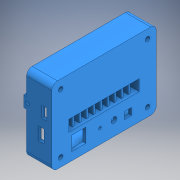
# Autodesk Inventor part: case_front
Saved by Autodesk Inventor 2016 (Build 200138000, 138)
## iProperties
Created: 2018-08-02
Part Number: case_front
Material: Generic
Document SubType Name: Modeling
Designer: Luke
Density: 1 g/cm^3
Appearance: Cyan
Author: Luke
Autodesk Inventor part; units mm, degrees
ref_plane "YZ Plane" through (0, 0, 0) normal (1, 0, 0) x (0, 1, 0)
ref_plane "XZ Plane" through (0, 0, 0) normal (0, 1, 0) x (-1, 0, 0)
ref_plane "XY Plane" through (0, 0, 0) normal (0, 0, 1) x (1, 0, 0)
sketch "Sketch1" plane through (0, 0, 0) normal (0, 1, 0) x (-1, 0, 0)
  line L0 (0, 0) -> (-74.5, 0)
  line L1 (-74.5, 0) -> (-74.5, 54.5)
  line L2 (-74.5, 54.5) -> (0, 54.5)
  line L3 (0, 54.5) -> (0, 0)
  dimension "d0" = 74.5
  dimension "d1" = 54.5
  constraints: 8 end point, 2 parallel, 1 horizontal, 1 perpendicular
  measures "d0" distance of L0.start L0.end
  measures "d1" distance of L0.end L1.end
extrude "Extrusion1" add sketch "Sketch1" along normal blind 2
ref_plane "Work Plane1" through (74.5, 0, 27.25) normal (0, 0, -1) x (-1, 0, 0)
ref_plane "Work Plane2" through (37.25, 0, 54.5) normal (1, 0, 0) x (0, 0, -1)
sketch "Sketch3" plane through (0, 2, 0) normal (0, 1, 0) x (1, 0, 0)
  line L0 (37.25, 10.9) -> (37.25, -65.4) construction
  line L1 (-14.9, -27.25) -> (89.4, -27.25) construction
  circle A0 centre (6.25, -6.25) radius 1.6
  circle A1 centre (68.25, -6.25) radius 1.6
  circle A2 centre (68.25, -48.25) radius 1.6
  circle A3 centre (6.25, -48.25) radius 1.6
  line L2 (6.25, -6.25) -> (68.25, -6.25) construction
  line L3 (68.25, -6.25) -> (68.25, -48.25) construction
  line L4 (68.25, -48.25) -> (6.25, -48.25) construction
  line L5 (6.25, -48.25) -> (6.25, -6.25) construction
  point P0 (0, 0)
  dimension "d4" = 3.2
  dimension "d5" = 3.2
  dimension "d6" = 3.2
  dimension "d7" = 3.2
  dimension "d8" = 62
  dimension "d9" = 42
  constraints: 8 end point, 4 centre point, 4 coincident, 2 parallel, 1 horizontal, 1 perpendicular, 2 other
  measures "d4" diameter of A0
  measures "d5" diameter of A1
  measures "d6" diameter of A2
  measures "d7" diameter of A3
  measures "d8" distance of L2.start L2.end
  measures "d9" distance of L2.end L3.end
extrude "Extrusion2" cut sketch "Sketch3" against normal up to surface (2 mm away)
sketch "Sketch4" plane through (0, 0, 0) normal (0, -1, 0) x (1, 0, 0)
  line L0 (0, 0) -> (74.5, 0) projected
  line L1 (74.5, 0) -> (74.5, 54.5) projected
  line L2 (74.5, 54.5) -> (0, 54.5) projected
  line L3 (0, 54.5) -> (0, 0) projected
  line L4 (72.5, 2) -> (2, 2)
  line L5 (2, 2) -> (2, 52.5)
  line L6 (2, 52.5) -> (72.5, 52.5)
  line L7 (72.5, 52.5) -> (72.5, 2)
  dimension "d12" = 2
  constraints: 8 end point, 3 other
  measures "d12" distance between parallel lines of L4 L0
extrude "Extrusion3" add sketch "Sketch4" along normal blind 16
sketch "Sketch5" plane through (0, 2, 0) normal (0, 1, 0) x (1, 0, 0)
  circle A0 centre (6.25, -48.25) radius 1.6 construction
  line L0 (14.175, -38.675) -> (24.175, -38.675)
  line L1 (24.175, -38.675) -> (24.175, -48.675)
  line L2 (24.175, -48.675) -> (14.175, -48.675)
  line L3 (14.175, -48.675) -> (14.175, -38.675)
  point P0 (0, 0)
  dimension "d15" = 7.925
  dimension "d16" = 10
  dimension "d17" = 10
  dimension "d18" = 9.575
  constraints: 8 end point, 2 parallel, 1 horizontal, 1 perpendicular
  measures "d15" distance from line of A0.centre L3
  measures "d16" distance of L1.end L2.end
  measures "d17" distance of L0.end L1.end
  measures "d18" distance from line of A0.centre L0
extrude "Extrusion4" cut sketch "Sketch5" against normal up to surface (2 mm away)
sketch "Sketch6" plane through (0, 2, 0) normal (-1, 0, 0) x (0, 0, 1)
  line L0 (16.5, -3.5) -> (24.5, -3.5)
  line L1 (24.5, -3.5) -> (24.5, -7)
  line L2 (24.5, -7) -> (16.5, -7)
  line L3 (16.5, -7) -> (16.5, -3.5)
  line L4 (0, 0) -> (54.5, 0) construction
  line L5 (54.5, 0) -> (54.5, -18) construction
  point P0 (0, -2)
  dimension "d21" = 30
  dimension "d22" = 3.5
  dimension "d23" = 8
  dimension "d24" = 3.5
  constraints: 8 end point, 2 parallel, 1 horizontal, 1 perpendicular
  measures "d21" distance between parallel lines of L5 L1
  measures "d22" distance of L0.end L1.end
  measures "d23" distance of L0.start L0.end
  measures "d24" distance between parallel lines of L0 L4
extrude "Extrusion5" cut sketch "Sketch6" against normal up to surface (2 mm away)
sketch "Sketch7" plane through (0, 2, 0) normal (-1, 0, 0) x (0, 0, 1)
  line L0 (0, 0) -> (54.5, 0) construction
  line L1 (54.5, 0) -> (54.5, -18) construction
  line L2 (30.5, -5.5) -> (39.5, -5.5)
  line L3 (39.5, -5.5) -> (39.5, -9.5)
  line L4 (39.5, -9.5) -> (30.5, -9.5)
  line L5 (30.5, -9.5) -> (30.5, -5.5)
  point P0 (0, -2)
  dimension "d27" = 15
  dimension "d28" = 9
  dimension "d29" = 4
  dimension "d30" = 5.5
  constraints: 8 end point, 2 parallel, 1 horizontal, 1 perpendicular
  measures "d27" distance between parallel lines of L1 L3
  measures "d28" distance of L2.start L2.end
  measures "d29" distance of L4.end L2.start
  measures "d30" distance between parallel lines of L2 L0
extrude "Extrusion6" cut sketch "Sketch7" against normal up to surface (2 mm away)
fillet "Fillet1" radius 4 8 edges at (72.5, -8, 52.5) (74.5, -7, 54.5) (72.5, -8, 2) (74.5, -7, 0) (2, -8, 2) (0, -7, 0) (0, -7, 54.5) (2, -8, 52.5)
sketch "Sketch8" plane through (0, -16, 50.5) normal (-1, 0, 0) x (0, 0, 1)
  line L0 (-50.5, 18) -> (-50.5, 0) construction
  line L1 (0, 0) -> (-46.5, 0) construction
  line L2 (-2, 0) -> (-44.5, 0) projected
  line L3 (-26, 0) -> (-34, 0)
  line L4 (-34, 0) -> (-34, -2)
  line L5 (-34, -2) -> (-26, -2)
  line L6 (-26, -2) -> (-26, 0)
  line L7 (-30, -2) -> (-30, 0) construction
  point P0 (-50.5, 16)
  dimension "d34" = 20.5
  dimension "d35" = 8
  dimension "d36" = 2
  constraints: 10 end point, 2 midpoint, 2 parallel, 1 horizontal, 1 perpendicular, 1 point on line
  measures "d34" distance between parallel lines of L0 L7
  measures "d35" distance of L4.end L5.end
  measures "d36" distance of L3.end L4.end
extrude "Extrusion7" add sketch "Sketch8" against normal up to surface (2 mm away)
sketch "Sketch9" plane through (0, -16, 50.5) normal (-1, 0, 0) x (0, 0, 1)
  line L0 (0, 0) -> (-26, 0) construction
  line L1 (-50.5, 18) -> (-50.5, 0) construction
  circle A0 centre (-30, 0.75) radius 1.25
  point P0 (-50.5, 16)
  dimension "d39" = 2.5
  dimension "d43" = 0.75
  dimension "d44" = 20.5
  constraints: 1 centre point
  measures "d39" diameter of A0
  measures "d43" distance from line of A0.centre L0
  measures "d44" distance from line of L1 A0.centre
extrude "Extrusion8" cut sketch "Sketch9" against normal up to surface (2 mm away)
sketch "Sketch10" plane through (0, 2, 0) normal (0, 1, 0) x (1, 0, 0)
  circle A0 centre (6.25, -48.25) radius 1.6 projected
  circle A1 centre (68.25, -48.25) radius 1.6 projected
  line L0 (12.25, -27.75) -> (62.25, -27.75)
  line L1 (62.25, -27.75) -> (62.25, -35.75)
  line L2 (62.25, -35.75) -> (12.25, -35.75)
  line L3 (12.25, -35.75) -> (12.25, -27.75)
  line L4 (6.25, -48.25) -> (68.25, -48.25) construction
  line L5 (37.25, -48.25) -> (37.25, -35.75) construction
  point P0 (0, 0)
  dimension "d45" = 12.5
  dimension "d46" = 8
  dimension "d47" = 50
  constraints: 12 end point, 2 horizontal, 2 midpoint, 2 parallel, 2 perpendicular
  measures "d45" distance from line of L4.start L2
  measures "d46" distance of L2.end L0.start
  measures "d47" distance of L0.start L0.end
extrude "Extrusion9" cut sketch "Sketch10" against normal up to surface (2 mm away) contours L0 L1 L2 L3
sketch "Sketch11" plane through (0, 0, 0) normal (0, -1, 0) x (1, 0, 0)
  line L0 (62.25, 27.75) -> (12.25, 27.75) projected
  line L1 (12.25, 27.75) -> (12.25, 35.75) projected
  line L2 (12.25, 35.75) -> (62.25, 35.75) projected
  line L3 (62.25, 35.75) -> (62.25, 27.75) projected
  line L4 (63.75, 37.25) -> (10.75, 37.25)
  line L5 (10.75, 37.25) -> (10.75, 26.25)
  line L6 (10.75, 26.25) -> (63.75, 26.25)
  line L7 (63.75, 26.25) -> (63.75, 37.25)
  point P0 (0, 0)
  dimension "d50" = 1.5
  constraints: 8 end point, 3 other
  measures "d50" distance between parallel lines of L2 L4
extrude "Extrusion10" add sketch "Sketch11" along normal blind 6
sketch "Sketch12" plane through (0, -6, 0) normal (0, -1, 0) x (1, 0, 0)
  line L0 (12.25, 27.75) -> (12.25, 35.75) projected
  line L1 (12.25, 35.75) -> (62.25, 35.75) projected
  line L2 (62.25, 35.75) -> (62.25, 27.75) projected
  line L3 (62.25, 27.75) -> (12.25, 27.75) projected
  line L4 (63.75, 37.25) -> (10.75, 37.25) projected
  line L5 (10.75, 37.25) -> (10.75, 26.25) projected
  line L6 (10.75, 26.25) -> (63.75, 26.25) projected
  line L7 (63.75, 26.25) -> (63.75, 37.25) projected
  line L8 (62.25, 35.75) -> (12.25, 35.75) construction
  line L9 (37.25, 35.75) -> (37.25, 27.75) construction
  line L10 (36.5, 35.75) -> (36.5, 27.75)
  line L11 (12.25, 27.75) -> (62.25, 27.75) projected
  line L12 (38, 35.75) -> (38, 27.75)
  line L13 (36.5, 35.75) -> (38, 35.75)
  line L14 (36.5, 27.75) -> (38, 27.75)
  point P0 (0, 0)
  dimension "d53" = 1.5
  constraints: 10 end point, 4 point on line, 2 collinear, 2 midpoint, 1 perpendicular, 1 vertical, 1 other
  measures "d53" distance between parallel lines of L12 L10
extrude "Extrusion11" add sketch "Sketch12" against normal blind 6 contours L10 L1 L12 L3
pattern_linear "Rectangular Pattern1" count 9 spacing 5 along (1, 0, 0) of "Extrusion11" first direction both ways yes
sketch "Sketch13" plane through (0, 2, 0) normal (0, 1, 0) x (1, 0, 0)
  circle A0 centre (68.25, -48.25) radius 1.6 construction
  line L0 (51.75, -42.75) -> (56.75, -42.75)
  line L1 (56.75, -42.75) -> (56.75, -47.75)
  line L2 (56.75, -47.75) -> (51.75, -47.75)
  line L3 (51.75, -47.75) -> (51.75, -42.75)
  line L4 (54.25, -42.75) -> (54.25, -47.75) construction
  line L5 (56.75, -45.25) -> (51.75, -45.25) construction
  point P0 (0, 0)
  point P1 (54.25, -45.25)
  dimension "d59" = 14
  dimension "d60" = 3
  dimension "d61" = 5
  dimension "d62" = 5
  constraints: 12 end point, 5 midpoint, 2 parallel, 1 horizontal, 1 perpendicular
  measures "d59" horizontal distance of A0.centre point (54.25, -45.25)
  measures "d60" vertical distance of A0.centre point (54.25, -45.25)
  measures "d61" distance of L2.end L0.start
  measures "d62" distance of L0.start L0.end
extrude "Extrusion12" cut sketch "Sketch13" against normal up to surface (2 mm away)
sketch "Sketch14" plane through (0, 2, 0) normal (0, 1, 0) x (1, 0, 0)
  circle A0 centre (6.25, -48.25) radius 1.6 construction
  circle A1 centre (34.25, -44.25) radius 1
  point P0 (0, 0)
  dimension "d65" = 2
  dimension "d66" = 28
  dimension "d67" = 4
  constraints: 1 centre point
  measures "d65" diameter of A1
  measures "d66" horizontal distance of A1.centre A0.centre
  measures "d67" vertical distance of A0.centre A1.centre
extrude "Extrusion13" cut sketch "Sketch14" against normal up to surface (2 mm away)
sketch "Sketch15" plane through (0, 2, 0) normal (0, 1, 0) x (1, 0, 0)
  circle A0 centre (6.25, -48.25) radius 1.6 construction
  circle A1 centre (44.25, -44.25) radius 2
  point P0 (0, 0)
  dimension "d70" = 38
  dimension "d71" = 4
  dimension "d72" = 4
  constraints: 1 centre point
  measures "d70" horizontal distance of A1.centre A0.centre
  measures "d71" vertical distance of A0.centre A1.centre
  measures "d72" diameter of A1
extrude "Extrusion14" cut sketch "Sketch15" against normal up to surface (2 mm away)
equation "\"d5\" = d4"
equation "\"d6\" = d5"
equation "\"d7\" = d6"
body "Solid1"
